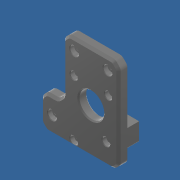
# Autodesk Inventor part: Print_Parts_F
Saved by Autodesk Inventor 2020 (Build 240168000, 168)
## iProperties
Created: 2020-09-26
Part Number: Print_Parts_F
Material: PC/ABS プラスチック
Document SubType Name: Modeling
Designer: kenta iguchi
Density: 0.357273 g/cm^3
Appearance: 滑らか - 黒
Author: kenta iguchi
Autodesk Inventor part; units mm, degrees
ref_plane "YZ Plane" through (0, 0, 0) normal (1, 0, 0) x (0, 1, 0)
ref_plane "XZ Plane" through (0, 0, 0) normal (0, 1, 0) x (-1, 0, 0)
ref_plane "XY Plane" through (0, 0, 0) normal (0, 0, 1) x (1, 0, 0)
sketch "スケッチ1" plane through (0, 0, 0) normal (0, 0, 1) x (1, 0, 0)
  line L0 (0, 0) -> (-50, 0)
  line L1 (-50, 0) -> (-50, -85)
  line L2 (-50, -85) -> (0, -85)
  line L3 (0, -85) -> (0, 0)
  dimension "d0" = 50
  dimension "d1" = 85
  constraints: 8 end point, 2 parallel, 1 horizontal, 1 perpendicular
  measures "d0" distance of L2.end L1.end
  measures "d1" distance of L1.end L0.end
extrude "押し出し1" add sketch "スケッチ1" along normal blind 8
sketch "スケッチ2" plane through (0, 0, 8) normal (0, 0, 1) x (1, 0, 0)
  line L0 (0, -85) -> (0, 0) projected
  line L1 (0, 0) -> (-50, 0) projected
  circle A0 centre (-25, -45) radius 11.15
  dimension "d4" = 45
  dimension "d5" = 25
  dimension "d6" = 22.3
  constraints: 1 centre point
  measures "d4" distance from line of A0.centre L1
  measures "d5" distance from line of L0 A0.centre
  measures "d6" diameter of A0
extrude "押し出し2" cut sketch "スケッチ2" against normal blind 10
sketch "スケッチ3" plane through (0, 0, 8) normal (0, 0, 1) x (1, 0, 0)
  circle A0 centre (-25, -45) radius 11.15 projected
  line L0 (-40.5, -60.5) -> (-9.5, -60.5)
  line L1 (-9.5, -60.5) -> (-9.5, -29.5)
  line L2 (-9.5, -29.5) -> (-40.5, -29.5)
  line L3 (-40.5, -29.5) -> (-40.5, -60.5)
  line L4 (-40.5, -60.5) -> (-9.5, -29.5) construction
  line L5 (-9.5, -60.5) -> (-40.5, -29.5) construction
  dimension "d9" = 31
  dimension "d10" = 31
  constraints: 12 end point, 2 midpoint, 2 parallel, 1 horizontal, 1 perpendicular
  measures "d9" distance of L2.end L1.end
  measures "d10" distance of L1.end L0.end
hole "穴1" at (-40.5, -29.5, 8) at (-9.5, -29.5, 8) direction (0, 0, -1) diameter 3.3 depth 58 counterbore diameter 6.5 counterbore depth 4
sketch "スケッチ4" plane through (0, 0, 0) normal (0, 0, -1) x (-1, 0, 0)
  line L0 (0, -85) -> (0, 0) projected
  line L1 (50, -85) -> (0, -85) projected
  point P0 (9.5, -80)
  point P1 (38.5, -66.5)
  dimension "d18" = 38.5
  dimension "d19" = 9.5
  dimension "d20" = 5
  dimension "d34" = 13.5
  measures "d18" distance from line of point (38.5, -66.5) L0
  measures "d19" distance from line of L0 point (9.5, -80)
  measures "d20" distance from line of point (9.5, -80) L1
  measures "d34" vertical distance of point (9.5, -80) point (38.5, -66.5)
hole "穴2" at (-9.5, -80, 0) at (-38.5, -66.5, 0) direction (0, 0, 1) diameter 3.3 depth 58
sketch "スケッチ8" plane through (0, 0, 0) normal (0, 0, -1) x (-1, 0, 0)
  circle A0 centre (38.5, -66.5) radius 1.65 projected
  line L0 (50, 0) -> (50, -85) projected
  line L1 (50, -85) -> (0, -85) projected
  line L2 (50, 0) -> (50, -85) projected
  line L3 (50, -54) -> (30.5, -54)
  line L4 (30.5, -54) -> (30.5, -70.5)
  line L5 (30.5, -70.5) -> (50, -70.5)
  line L6 (50, -70.5) -> (50, -54)
  circle A1 centre (38.5, -66.5) radius 8
  circle A2 centre (38.5, -66.5) radius 6
  circle A3 centre (38.5, -66.5) radius 4
  circle A4 centre (9.5, -80) radius 1.65 projected
  circle A5 centre (38.5, -66.5) radius 1.65 projected
  circle A6 centre (40.5, -29.5) radius 1.65 projected
  circle A7 centre (9.5, -29.5) radius 1.65 projected
  circle A8 centre (25, -45) radius 11.15 projected
  line L7 (50, 0) -> (50, -85) projected
  line L8 (0, 0) -> (50, 0) projected
  line L9 (0, -85) -> (0, 0) projected
  line L10 (50, -85) -> (0, -85) projected
  point P0 (31.582, -54)
  point P1 (30.5, -54.6991)
  dimension "d35" = 31
  dimension "d36" = 16
  dimension "d37" = 12
  dimension "d38" = 2
  constraints: 8 end point, 3 centre point, 2 coincident, 2 parallel, 2 tangent, 1 horizontal, 1 perpendicular, 1 point on line
  measures "d35" distance between parallel lines of L3 L1
  measures "d36" diameter of A1
  measures "d37" diameter of A2
  measures "d38" radial gap between concentric circles of A2 A3
extrude "押し出し5" add sketch "スケッチ8" along normal blind 10 contours L0 L5 A1 L4 A8 L3 | L5 A2 A1 | A3 | L5 A2 | L5 L4 A1 picked at (45.7558, -65.8618) picked at (43.741, -67.2784)
sketch "スケッチ9" plane through (0, 0, -10) normal (0, 0, -1) x (-1, 0, 0)
  line L0 (50, -54) -> (31.582, -54) projected
  circle A0 centre (38.5, -66.5) radius 1.65 projected
  circle A1 centre (38.5, -66.5) radius 10
  line L1 (50, -70.5) -> (36.15, -70.5)
  line L2 (36.15, -70.5) -> (36.15, -54)
  line L3 (36.15, -54) -> (50, -54)
  line L4 (50, -54) -> (50, -70.5)
  line L5 (30.5, -54.6991) -> (30.5, -70.5) projected
  line L6 (38.5, -56.5) -> (21.3308, -56.5)
  point P0 (30.5, -54)
  point P1 (0, 0)
  point P2 (36.15, -56.78)
  point P3 (47.6652, -70.5)
  point P4 (36.15, -56.5)
  dimension "d41" = 20
  dimension "d42" = 13.85
  constraints: 10 end point, 2 parallel, 2 perpendicular, 1 coincident, 1 horizontal, 1 point on line, 1 vertical alignment, 3 other
  measures "d42" distance of L2.end L3.end
extrude "押し出し6" add sketch "スケッチ9" along normal blind 10 contours L4 L1 A1 L6 L2 L0
sketch "スケッチ10" plane through (0, 0, 8) normal (0, 0, 1) x (1, 0, 0)
  line L0 (0, -85) -> (0, 0) projected
  line L1 (0, -85) -> (20, -85)
  line L2 (20, -85) -> (20, -55)
  line L3 (20, -55) -> (0, -55)
  line L4 (0, -55) -> (0, -85)
  dimension "d48" = 20
  dimension "d49" = 30
  constraints: 8 end point, 2 parallel, 1 horizontal, 1 perpendicular
  measures "d48" distance of L3.end L2.end
  measures "d49" distance of L2.end L1.end
extrude "押し出し7" add sketch "スケッチ10" against normal up to surface (8 mm away)
chamfer "面取り2" distance 5 angle 45 6 edges at (-50, -85, 4) (20, -85, 4) (20, -55, 4) (0, -55, 4) (0, 0, 4) (-50, 0, 4)
fillet "フィレット1" radius 5 12 edges at (-50, -80, 4) (-45, -85, 4) (15, -85, 4) (20, -80, 4) (20, -60, 4) (15, -55, 4) (5, -55, 4) (0, -50, 4) (0, -5, 4) (-5, 0, 4) (-45, 0, 4) (-50, -5, 4)
sketch "スケッチ21" plane through (0, 0, -20) normal (0, 0, -1) x (-1, 0, 0)
  line L0 (47.6652, -70.5) -> (50, -70.5) projected
  arc A0 (47.6652, -70.5) -> (38.5, -56.5) centre (38.5, -66.5) ccw projected
  line L1 (47.6652, -70.5) -> (48.5, -70.5)
  line L2 (48.5, -70.5) -> (48.5, -66.5)
  line L3 (48.5, -66.5) -> (47.6652, -66.5)
  line L4 (47.6652, -66.5) -> (47.6652, -70.5)
  point P0 (0, 0)
  constraints: 8 end point, 2 parallel, 1 horizontal, 1 perpendicular, 1 point on circle
extrude "押し出し16" cut sketch "スケッチ21" against normal up to surface (10 mm away)
sketch "スケッチ11" plane through (0, 0, -10) normal (0, 0, -1) x (-1, 0, 0)
  line L0 (36.15, -56.5) -> (36.15, -54) projected
  line L1 (36.15, -54) -> (31.582, -54) projected
  arc A0 (30.5, -54.6991) -> (31.582, -54) centre (25, -45) ccw projected
  line L2 (30.5, -54.6991) -> (30.5, -70.5) projected
  line L3 (36.15, -56.5) -> (28.5102, -56.5)
  line L4 (28.5102, -56.5) -> (28.5102, -54)
  line L5 (28.5102, -54) -> (36.15, -54)
  line L6 (36.15, -54) -> (36.15, -56.5)
  point P0 (0, 0)
  point P1 (30.5, -56.5)
  constraints: 8 end point, 2 parallel, 1 horizontal, 1 horizontal alignment, 1 perpendicular
extrude "押し出し8" cut sketch "スケッチ11" against normal up to surface (10 mm away) contours L3 L2 A0 L1 L0
chamfer "面取り10" distance 2.5 angle 45 1 edges at (-36.15, -56.5, -5)
sketch "スケッチ22" plane through (0, 0, -10) normal (0, 0, -1) x (-1, 0, 0)
  line L0 (33.65, -56.5) -> (30.5, -56.5) projected
  line L1 (30.5, -56.5) -> (30.5, -70.5) projected
  line L2 (36.15, -54) -> (33.65, -56.5) projected
  line L3 (33.65, -56.5) -> (19.9925, -70.1575)
  point P0 (0, 0)
  point P1 (30.5, -59.65)
  constraints: 2 end point, 1 collinear
extrude "押し出し17" cut sketch "スケッチ22" against normal up to surface (10 mm away)
sketch "スケッチ12" plane through (0, 0, -10) normal (0, 0, -1) x (-1, 0, 0)
  circle A0 centre (38.5, -66.5) radius 1.65 projected
  circle A1 centre (38.5, -66.5) radius 1.65 projected
  circle A2 centre (38.5, -66.5) radius 3
  point P0 (0, 0)
  dimension "d64" = 6
  constraints: 1 centre point, 1 coincident
  measures "d64" diameter of A2
extrude "押し出し9" add sketch "スケッチ12" along normal blind 0.5
chamfer "面取り5" distance 0.5 angle 45 1 edges at (-35.5, -66.5, -10)
sketch "スケッチ13" plane through (0, 0, 0) normal (0, 0, -1) x (-1, 0, 0)
  circle A0 centre (9.5, -80) radius 1.65 projected
  circle A1 centre (9.5, -80) radius 3
  point P0 (0, 0)
  dimension "d70" = 6
  constraints: 1 centre point, 1 coincident
  measures "d70" diameter of A1
extrude "押し出し10" add sketch "スケッチ13" along normal blind 1
chamfer "面取り6" distance 1 angle 45 1 edges at (-6.5, -80, 0)
fillet "フィレット2" radius 1.5 1 edges at (-50, -70.5, -10)
mirror "Mirror1" about plane through (-50, 0, 0) normal (-1, 0, 0) remove original yes
sketch "Sketch14" plane through (-50, -54, -20) normal (0, 0, -1) x (-1, 0, 0)
  arc A0 (11.5, -2.5) -> (1.5, -12.5) centre (11.5, -12.5) ccw projected
  arc A1 (0, -15) -> (1.5, -16.5) centre (1.5, -15) ccw projected
  arc A2 (11.5, -2.5) -> (1.5, -12.5) centre (11.5, -12.5) ccw projected
  line L0 (13.85, -2.5) -> (11.5, -2.5) projected
  line L1 (13.85, 0) -> (13.85, -2.5) projected
  line L2 (0, 0) -> (13.85, 0) projected
  line L3 (0, -15) -> (0, 0) projected
  line L4 (13.85, 0) -> (13.85, -2.5) projected
  line L5 (11.5, -2.5) -> (13.85, -2.5) projected
  arc A3 (11.5, -2.5) -> (1.5, -12.5) centre (11.5, -12.5) ccw projected
  line L6 (19.5, -5.65) -> (19.5, -16.5) projected
  circle A4 centre (11.5, -12.5) radius 3.5 projected
  line L7 (13.85, 0) -> (19.5, -5.65) projected
  line L8 (1.5, -12.5) -> (1.5, -16.5) projected
  line L9 (19.5, -16.5) -> (1.5, -16.5) projected
  line L10 (1.5, -12.5) -> (1.5, -16.5) projected
  point P0 (-50, 54)
  point P1 (3.4377, -16.5)
  point P2 (11.5, -2.5)
  point P3 (1.5, -16.5)
  point P4 (11.5, -2.5)
  point P5 (2.3348, -16.5)
  point P6 (3.4377, -16.5)
  point P7 (1.5, -16.5)
extrude "Extrusion11" cut sketch "Sketch14" against normal up to surface (20 mm away) contours L0 L1 L7 L6 L9 L8 A0 | A4
sketch "Sketch15" plane through (-50, -54, -20) normal (0, 0, -1) x (-1, 0, 0)
  arc A0 (0, -15) -> (1.5, -16.5) centre (1.5, -15) ccw projected
  arc A1 (11.5, -2.5) -> (1.5, -12.5) centre (11.5, -12.5) ccw projected
  line L0 (13.85, -2.5) -> (11.5, -2.5) projected
  line L1 (13.85, 0) -> (13.85, -2.5) projected
  line L2 (0, 0) -> (13.85, 0) projected
  line L3 (0, -15) -> (0, 0) projected
  line L4 (1.5, -12.5) -> (1.5, -16.5) projected
  point P0 (-50, 54)
extrude "Extrusion12" cut sketch "Sketch15" against normal blind 9.5
sketch "Sketch16" plane through (-57.0711, 0, 0) normal (0, 0, -1) x (-1, 0, 0)
  circle A0 centre (33.4289, -29.5) radius 1.65 projected
  circle A1 centre (2.4289, -29.5) radius 1.65 projected
  circle A2 centre (17.9289, -45) radius 11.15 projected
  arc A3 (-7.0711, -69) -> (-5.5711, -70.5) centre (-5.5711, -69) ccw projected
  line L0 (-7.0711, -69) -> (-7.0711, -77.9289) projected
  arc A4 (-7.0711, -77.9289) -> (-5.6066, -81.4645) centre (-2.0711, -77.9289) ccw projected
  line L1 (-5.6066, -81.4645) -> (-3.5355, -83.5355) projected
  arc A5 (-3.5355, -83.5355) -> (0, -85) centre (0, -80) ccw projected
  line L2 (0, -85) -> (55.8579, -85) projected
  arc A6 (55.8579, -85) -> (59.3934, -83.5355) centre (55.8579, -80) ccw projected
  line L3 (59.3934, -83.5355) -> (61.4645, -81.4645) projected
  arc A7 (61.4645, -81.4645) -> (62.9289, -77.9289) centre (57.9289, -77.9289) ccw projected
  line L4 (62.9289, -62.0711) -> (62.9289, -77.9289) projected
  arc A8 (62.9289, -62.0711) -> (61.4645, -58.5355) centre (57.9289, -62.0711) ccw projected
  line L5 (61.4645, -58.5355) -> (59.3934, -56.4645) projected
  arc A9 (59.3934, -56.4645) -> (55.8579, -55) centre (55.8579, -60) ccw projected
  line L6 (50, -55) -> (55.8579, -55) projected
  arc A10 (46.4645, -53.5355) -> (50, -55) centre (50, -50) ccw projected
  line L7 (46.4645, -53.5355) -> (44.3934, -51.4645) projected
  arc A11 (42.9289, -47.9289) -> (44.3934, -51.4645) centre (47.9289, -47.9289) ccw projected
  line L8 (42.9289, -47.9289) -> (42.9289, -7.0711) projected
  arc A12 (42.9289, -7.0711) -> (41.4645, -3.5355) centre (37.9289, -7.0711) ccw projected
  line L9 (41.4645, -3.5355) -> (39.3934, -1.4645) projected
  arc A13 (39.3934, -1.4645) -> (35.8579, 0) centre (35.8579, -5) ccw projected
  line L10 (35.8579, 0) -> (0, 0) projected
  arc A14 (0, 0) -> (-3.5355, -1.4645) centre (0, -5) ccw projected
  line L11 (-3.5355, -1.4645) -> (-5.6066, -3.5355) projected
  arc A15 (-5.6066, -3.5355) -> (-7.0711, -7.0711) centre (-2.0711, -7.0711) ccw projected
  line L12 (-7.0711, -7.0711) -> (-7.0711, -54) projected
  line L13 (6.7789, -54) -> (-7.0711, -54) projected
  circle A16 centre (33.4289, -80) radius 4 projected
  circle A17 centre (4.4289, -66.5) radius 3
  line L14 (6.7789, -54) -> (6.7789, -56.5) projected
  line L15 (6.7789, -56.5) -> (4.4289, -56.5) projected
  arc A18 (4.4289, -56.5) -> (-5.5711, -66.5) centre (4.4289, -66.5) ccw projected
  circle A19 centre (4.4289, -66.5) radius 1.65 projected
  line L16 (-5.5711, -66.5) -> (-5.5711, -70.5) projected
  point P0 (-57.0711, 0)
  dimension "d81" = 6
  constraints: 1 centre point
  measures "d81" diameter of A17
extrude "Extrusion13" add sketch "Sketch16" along normal blind 1 contours A17
chamfer "Chamfer7" distance 1 angle 45 1 edges at (-58.5, -66.5, 0)
sketch "スケッチ17" plane through (-112.9289, -55, 8) normal (0, 0, 1) x (1, 0, 0)
  line L0 (20, 55) -> (55.8579, 55) projected
  line L1 (12.9289, 7.0711) -> (12.9289, 47.9289) projected
  line L2 (-7.0711, -22.9289) -> (-7.0711, -7.0711) projected
  line L3 (55.8579, -30) -> (0, -30) projected
  line L4 (62.9289, 47.9289) -> (62.9289, -22.9289) projected
  point P0 (112.9289, 55)
  point P1 (52.9289, 45)
  point P2 (22.9289, 45)
  point P3 (2.9289, -15)
  dimension "d87" = 10
  dimension "d88" = 10
  dimension "d89" = 10
  dimension "d90" = 10
  dimension "d91" = 15
  constraints: 1 horizontal alignment
  measures "d87" distance from line of point (52.929, 45) L0
  measures "d88" distance from line of point (52.929, 45) L4
  measures "d89" distance from line of L1 point (22.929, 45)
  measures "d90" distance from line of L2 point (2.929, -15)
  measures "d91" distance from line of point (2.929, -15) L3
hole "穴3" at (-60, -10, 8) at (-90, -10, 8) at (-110, -70, 8) direction (0, 0, -1) diameter 4.3 end through all counterbore diameter 8 counterbore depth 4
chamfer "面取り8" distance 2 angle 45 24 edges at (-50, -42.5, 8) (-50.3806, -79.8423, 8) (-52.5, -82.5, 8) (-55.1577, -84.6194, 8) (-85, -85, 8) (-114.8423, -84.6194, 8) (-117.5, -82.5, 8) (-119.6194, -79.8423, 8) (-120, -70, 8) (-119.6194, -60.1577, 8) (-117.5, -57.5, 8) (-114.8423, -55.3806, 8) (-110, -55, 8) (-105.1577, -54.6194, 8) (-102.5, -52.5, 8) (-100.3806, -49.8423, 8) (-100, -27.5, 8) (-99.6194, -5.1577, 8) (-97.5, -2.5, 8) (-94.8423, -0.3806, 8) (-75, 0, 8) (-55.1577, -0.3806, 8) (-52.5, -2.5, 8) (-50.3806, -5.1577, 8)
sketch "スケッチ18" plane through (-112.9289, -83, 8) normal (0, 0, 1) x (1, 0, 0)
  circle A0 centre (51.4289, 16.5) radius 1.65 projected
  circle A1 centre (22.4289, 3) radius 1.65 projected
  point P0 (112.9289, 83)
hole "穴4" at (-61.5, -66.5, 8) at (-90.5, -80, 8) direction (0, 0, -1) diameter 7 depth 4
sketch "スケッチ19" plane through (-61.5, -66.5, 4) normal (0, 0, 1) x (1, 0, 0)
  circle A0 centre (0, 0) radius 3.5 projected
  circle A1 centre (2, 37) radius 3.25 projected
  circle A2 centre (2, 37) radius 1.65 projected
  circle A3 centre (1.5, 56.5) radius 4 projected
  circle A4 centre (-28.5, 56.5) radius 4 projected
  circle A5 centre (-28.5, 56.5) radius 2.15 projected
  circle A6 centre (-29, 37) radius 3.25 projected
  circle A7 centre (-29, 37) radius 1.65 projected
  circle A8 centre (-48.5, -3.5) radius 4 projected
  circle A9 centre (-48.5, -3.5) radius 2.15 projected
  circle A10 centre (-29, -13.5) radius 1.65 projected
  circle A11 centre (-29, -13.5) radius 3.5 projected
  line L0 (1.65, 1.65) -> (-1.65, 1.65)
  line L1 (-1.65, 1.65) -> (-1.65, -1.65)
  line L2 (-1.65, -1.65) -> (1.65, -1.65)
  line L3 (1.65, -1.65) -> (1.65, 1.65)
  line L4 (1.65, 1.65) -> (-1.65, -1.65) construction
  line L5 (-1.65, 1.65) -> (1.65, -1.65) construction
  line L6 (3.65, 38.65) -> (0.35, 38.65)
  line L7 (0.35, 38.65) -> (0.35, 35.35)
  line L8 (0.35, 35.35) -> (3.65, 35.35)
  line L9 (3.65, 35.35) -> (3.65, 38.65)
  line L10 (3.65, 38.65) -> (0.35, 35.35) construction
  line L11 (0.35, 38.65) -> (3.65, 35.35) construction
  line L12 (-0.65, 58.65) -> (3.65, 58.65)
  line L13 (3.65, 58.65) -> (3.65, 54.35)
  line L14 (3.65, 54.35) -> (-0.65, 54.35)
  line L15 (-0.65, 54.35) -> (-0.65, 58.65)
  line L16 (-0.65, 58.65) -> (3.65, 54.35) construction
  line L17 (3.65, 58.65) -> (-0.65, 54.35) construction
  line L18 (-26.35, 58.65) -> (-30.65, 58.65)
  line L19 (-30.65, 58.65) -> (-30.65, 54.35)
  line L20 (-30.65, 54.35) -> (-26.35, 54.35)
  line L21 (-26.35, 54.35) -> (-26.35, 58.65)
  circle A12 centre (-28.5, 56.5) radius 4 projected
  line L22 (-26.35, 58.65) -> (-30.65, 54.35) construction
  line L23 (-30.65, 58.65) -> (-26.35, 54.35) construction
  line L24 (-27.35, 38.65) -> (-30.65, 38.65)
  line L25 (-30.65, 38.65) -> (-30.65, 35.35)
  line L26 (-30.65, 35.35) -> (-27.35, 35.35)
  line L27 (-27.35, 35.35) -> (-27.35, 38.65)
  line L28 (-27.35, 38.65) -> (-30.65, 35.35) construction
  line L29 (-30.65, 38.65) -> (-27.35, 35.35) construction
  line L30 (-46.35, -1.35) -> (-50.65, -1.35)
  line L31 (-50.65, -1.35) -> (-50.65, -5.65)
  line L32 (-50.65, -5.65) -> (-46.35, -5.65)
  line L33 (-46.35, -5.65) -> (-46.35, -1.35)
  line L34 (-46.35, -1.35) -> (-50.65, -5.65) construction
  line L35 (-50.65, -1.35) -> (-46.35, -5.65) construction
  line L36 (-27.35, -11.85) -> (-30.65, -11.85)
  line L37 (-30.65, -11.85) -> (-30.65, -15.15)
  line L38 (-30.65, -15.15) -> (-27.35, -15.15)
  line L39 (-27.35, -15.15) -> (-27.35, -11.85)
  line L40 (-27.35, -11.85) -> (-30.65, -15.15) construction
  line L41 (-30.65, -11.85) -> (-27.35, -15.15) construction
  point P0 (61.5, 66.5)
  constraints: 84 end point, 14 midpoint, 14 parallel, 7 horizontal, 7 perpendicular, 5 point on line
extrude "押し出し14" cut sketch "スケッチ19" against normal blind 0.6 contours A2 | L9 L8 A2 | A2 L6 L9 | A2 L7 L6 | L8 L7 A2 | A5 | L21 L20 A5 | A5 L18 L21 | A5 L19 L18 | L20 L19 A5 | A7 | L27 L26 A7 | A7 L24 L27 | A7 L25 L24 | L26 L25 A7 | A9 | L33 L32 A9 | A9 L30 L33 | A9 L31 L30 | L32 L31 A9 | A10 | L39 L38 A10 | A10 L36 L39 | A10 L37 L36 | L38 L37 A10 | L3 L2 L1 L0 | L12 L13 L14 L15
sketch "スケッチ20" plane through (-61.5, -66.5, 4) normal (0, 0, 1) x (1, 0, 0)
  line L0 (-1.65, -1.65) -> (-1.65, 1.65) projected
  line L1 (1.65, 1.65) -> (1.65, -1.65) projected
  circle A0 centre (0, 0) radius 3.5 projected
  circle A1 centre (2, 37) radius 3.25 projected
  circle A2 centre (1.5, 56.5) radius 4 projected
  circle A3 centre (-28.5, 56.5) radius 4 projected
  circle A4 centre (-29, 37) radius 3.25 projected
  circle A5 centre (-48.5, -3.5) radius 4 projected
  line L2 (-30.65, -15.15) -> (-30.65, -11.85) projected
  line L3 (-30.65, -11.85) -> (-27.35, -11.85) projected
  line L4 (-27.35, -11.85) -> (-27.35, -15.15) projected
  line L5 (-27.35, -15.15) -> (-30.65, -15.15) projected
  circle A6 centre (-29, -13.5) radius 3.5 projected
  line L6 (1.65, 3.0867) -> (-1.65, 3.0867)
  line L7 (-1.65, 3.0867) -> (-1.65, -3.0867)
  line L8 (-1.65, -3.0867) -> (1.65, -3.0867)
  line L9 (1.65, -3.0867) -> (1.65, 3.0867)
  line L10 (1.65, 3.0867) -> (-1.65, -3.0867) construction
  line L11 (-1.65, 3.0867) -> (1.65, -3.0867) construction
  line L12 (3.65, 39.8) -> (0.35, 39.8)
  line L13 (0.35, 39.8) -> (0.35, 34.2)
  line L14 (0.35, 34.2) -> (3.65, 34.2)
  line L15 (3.65, 34.2) -> (3.65, 39.8)
  line L16 (3.65, 39.8) -> (0.35, 34.2) construction
  line L17 (0.35, 39.8) -> (3.65, 34.2) construction
  circle A7 centre (1.5, 56.5) radius 4 projected
  line L18 (3.65, 59.8731) -> (-0.65, 59.8731)
  line L19 (-0.65, 59.8731) -> (-0.65, 53.1269)
  line L20 (-0.65, 53.1269) -> (3.65, 53.1269)
  line L21 (3.65, 53.1269) -> (3.65, 59.8731)
  line L22 (3.65, 59.8731) -> (-0.65, 53.1269) construction
  line L23 (-0.65, 59.8731) -> (3.65, 53.1269) construction
  line L24 (-26.35, 59.8731) -> (-30.65, 59.8731)
  line L25 (-30.65, 59.8731) -> (-30.65, 53.1269)
  line L26 (-30.65, 53.1269) -> (-26.35, 53.1269)
  line L27 (-26.35, 53.1269) -> (-26.35, 59.8731)
  line L28 (-26.35, 59.8731) -> (-30.65, 53.1269) construction
  line L29 (-30.65, 59.8731) -> (-26.35, 53.1269) construction
  circle A8 centre (-29, 37) radius 3.25 projected
  line L30 (-27.35, 39.8) -> (-30.65, 39.8)
  line L31 (-30.65, 39.8) -> (-30.65, 34.2)
  line L32 (-30.65, 34.2) -> (-27.35, 34.2)
  line L33 (-27.35, 34.2) -> (-27.35, 39.8)
  line L34 (-27.35, 39.8) -> (-30.65, 34.2) construction
  line L35 (-30.65, 39.8) -> (-27.35, 34.2) construction
  circle A9 centre (-48.5, -3.5) radius 4 projected
  line L36 (-46.35, -0.1269) -> (-50.65, -0.1269)
  line L37 (-50.65, -0.1269) -> (-50.65, -6.8731)
  line L38 (-50.65, -6.8731) -> (-46.35, -6.8731)
  line L39 (-46.35, -6.8731) -> (-46.35, -0.1269)
  line L40 (-46.35, -0.1269) -> (-50.65, -6.8731) construction
  line L41 (-50.65, -0.1269) -> (-46.35, -6.8731) construction
  circle A10 centre (-29, -13.5) radius 3.5 projected
  line L42 (-27.35, -10.4133) -> (-30.65, -10.4133)
  line L43 (-30.65, -10.4133) -> (-30.65, -16.5867)
  line L44 (-30.65, -16.5867) -> (-27.35, -16.5867)
  line L45 (-27.35, -16.5867) -> (-27.35, -10.4133)
  line L46 (-27.35, -10.4133) -> (-30.65, -16.5867) construction
  line L47 (-30.65, -10.4133) -> (-27.35, -16.5867) construction
  circle A11 centre (-28.5, 56.5) radius 4 projected
  circle A12 centre (-29, 37) radius 3.25 projected
  circle A13 centre (-48.5, -3.5) radius 4 projected
  arc A14 (-27.1972, -16.5) -> (-30.8028, -16.5) centre (-29, -13.5) ccw projected
  circle A15 centre (0, 0) radius 3.5 projected
  circle A16 centre (2, 37) radius 3.25 projected
  circle A17 centre (1.5, 56.5) radius 4 projected
  point P0 (61.5, 66.5)
  point P1 (-26.35, 53.1269)
  point P2 (-26.35, 59.8731)
  point P3 (-30.65, 59.8731)
  point P4 (-30.65, 53.1269)
  point P5 (-46.35, -0.1269)
  point P6 (-50.65, -0.1269)
  point P7 (-50.65, -6.8731)
  point P8 (-46.35, -6.8731)
  point P9 (-27.35, -10.4133)
  point P10 (1.65, 3.0867)
  point P11 (-1.65, 3.0867)
  point P12 (1.65, -3.0867)
  point P13 (3.65, 39.8)
  point P14 (0.35, 39.8)
  point P15 (3.65, 39.8)
  point P16 (-26.35, 53.1269)
  point P17 (-30.65, 53.1269)
  point P18 (-30.65, 59.8731)
  point P19 (-26.35, 59.8731)
  point P20 (0.35, 38.65)
  point P21 (-0.65, 58.65)
  point P22 (-30.65, 58.65)
  point P23 (-30.65, 38.65)
  point P24 (-50.65, -1.35)
  constraints: 84 end point, 14 midpoint, 14 parallel, 10 point on circle, 7 horizontal, 7 perpendicular, 7 vertical alignment, 2 point on line, 6 other
extrude "押し出し15" cut sketch "スケッチ20" against normal blind 0.3 contours L0 L7 L6 L9 L1 L8 | L8 A0 | A0 L6 | L12 A1 | L15 L14 L13 L12 | A1 L14 | L18 A2 | L21 L20 L19 L18 | A2 L20 | L24 A3 | L27 L26 L25 L24 | A3 L26 | L30 A4 | L33 L32 L31 L30 | A4 L32 | L36 A5 | L39 L38 L37 L36 | A5 L38 | L2 L3 L4 L5 | L5 L45 L44 L43 | L43 L42 L45 L3 | L44 A6 | A6 L42
chamfer "面取り9" distance 0.5 angle 45 7 edges at (-110, -66, 8) (-90.5, -76.5, 8) (-61.5, -63, 8) (-59.5, -26.25, 8) (-90.5, -26.25, 8) (-90, -6, 8) (-60, -6, 8)
chamfer "面取り11" distance 1 angle 45 2 edges at (-63.85, -45, 8) (-63.85, -45, 0)
